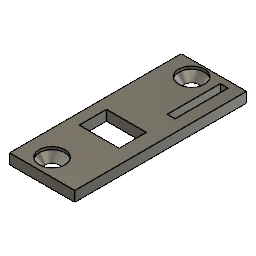
Super 8mm Focal Point v1 (Autodesk Fusion 360 design; units mm, degrees)
Autodesk Fusion 360 part; units mm, degrees
sketch "Sketch1" plane through (0, 0, 0) normal (0, 1, 0) x (1, 0, 0)
  line L0 (0, 0) -> (10.1, 0)
  line L1 (10.1, 0) -> (10.1, -26.54)
  line L2 (10.1, -26.54) -> (0, -26.54)
  line L3 (0, -26.54) -> (0, 0)
  line L4 (5.05, -17.44) -> (1.7, -17.44)
  line L5 (1.7, -17.44) -> (7.85, -17.44)
  line L6 (7.85, -17.44) -> (7.85, -13.24)
  line L7 (7.85, -13.24) -> (1.7, -13.24)
  line L8 (1.7, -13.24) -> (1.7, -17.44)
  line L9 (8.25, 0) -> (8.25, -1)
  line L10 (8.25, -1) -> (7.05, -1)
  line L11 (7.05, -1) -> (7.05, -9.2)
  line L12 (7.05, -9.2) -> (8.25, -9.2)
  line L13 (8.25, -9.2) -> (8.25, -1)
  circle A0 centre (3.9, -23.84) radius 1.1
  circle A1 centre (3.9, -2.3) radius 1.1
  dimension "d1" = 10.1
  dimension "d2" = 26.54
  dimension "d6" = 6.15
  dimension "d7" = 4.2
  dimension "d12" = 1.85
  dimension "d15" = 1
  dimension "d16" = 8.2
  dimension "d17" = 1.2
  dimension "d24" = 2.2
  dimension "d25" = 2.2
  constraint horizontal L0
  constraint vertical L1
  constraint vertical L3
  constraint coincident L0.start L3.end
  constraint horizontal L5
  constraint vertical L6
  constraint horizontal L7
  constraint vertical L8
  constraint horizontal L10
  constraint vertical L11
  constraint horizontal L12
  constraint vertical L13
  measures "d1" distance of L0.start L0.end
  measures "d2" distance of L0.start L2.end
  measures "d6" distance of L4.end L5.end
  measures "d7" distance of L4.end L7.end
  measures "d12" distance of L0.end L9.start
  measures "d15" distance of L9.start L9.end
  measures "d16" distance of L9.end L12.end
  measures "d17" distance of L9.end L10.end
  measures "d24" diameter of A0
  measures "d25" diameter of A1
extrude "Extrude1" add sketch "Sketch1" along normal blind 1.6
sketch "Sketch2" plane through (0, 0, 0) normal (0, 1, 0) x (1, 0, 0)
  circle A0 centre (3.9, -2.3) radius 2
  circle A1 centre (3.9, -23.84) radius 2
  point P0 (3.9, -2.3)
  point P1 (3.9, -23.84)
  dimension "d28" = 4
  dimension "d29" = 4
  constraint coincident P0 A0.centre
  constraint coincident P1 A1.centre
  measures "d28" diameter of A0
  measures "d29" diameter of A1
extrude "Extrude2" cut sketch "Sketch2" along normal blind 3 and the other way blind -1.2
fillet "Fillet1" radius 28.5 1 edges at (2.8744, 1.2, 2.6978)
fillet "Fillet2" radius 29 1 edges at (2.8744, 1.2, 24.2378)
